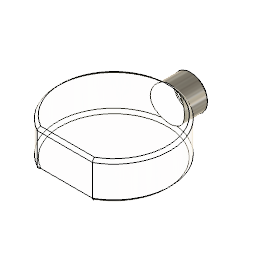
磁流体 (Autodesk Fusion 360 design; units mm, degrees)
part number: 2025-11-04-10-34-55-374
Autodesk Fusion 360 part; units mm, degrees
sketch "Sketch1" plane through (0, 0, 0) normal (0, 0, 1) x (1, 0, 0)
  circle A0 centre (0, 0) radius 40
  dimension "d1" = 80
  constraint coincident A0.centre origin
  measures "d1" diameter of A0
extrude "Extrude1" add sketch "Sketch1" along normal blind 26
sketch "Sketch2" plane through (0, 0, 0) normal (0, 1, 0) x (1, 0, 0)
  line L0 (-40, -26) -> (40, -26) construction
  line L1 (-40, 0) -> (40, 0) construction
  line L2 (0, 0) -> (0, -26) construction
  circle A0 centre (0, -13) radius 12.142
  constraint coincident L2.start origin
  constraint midpoint L0 L2.end
  constraint midpoint L2 A0.centre
extrude "Extrude2" add sketch "Sketch2" along normal blind 55
sketch "Sketch3" plane through (0, 0, 26) normal (0, 0, 1) x (-1, 0, 0)
  circle A0 centre (0, 0) radius 40
  line L0 (19.6984, 34.8134) -> (-19.6984, 34.8134)
  line L1 (19.6984, 34.8134) -> (19.6984, 40)
  line L2 (19.6984, 40) -> (-19.6984, 40)
  line L3 (-19.6984, 40) -> (-19.6984, 34.8134)
  constraint coincident A0 L0.start
  constraint coincident A0 L0.end
  constraint horizontal L0
  constraint perpendicular L0 L1
  constraint perpendicular L1 L2
  constraint perpendicular L0 L3
extrude "Extrude3" cut sketch "Sketch3" against normal blind 50 contours A0 L0 picked at (1.7116, 36.432)
fillet "Fillet1" radius 2 2 edges at (0, 40, 26) (0, -34.8134, 26)
fillet "Fillet2" radius 2 2 edges at (0, 40, 0) (0, -34.8134, 0)
fillet "Fillet3" radius 0.5 1 edges at (-11.3203, 55, 17.3907)
